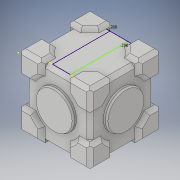
# Autodesk Inventor part: CapStone
Saved by Autodesk Inventor 2018 (Build 220112000, 112)
## iProperties
Created: 2020-01-09
Part Number: CapStone
Material: Generic
Document SubType Name: Modeling
Designer: AOFUser
Density: 1 g/cm^3
Appearance: Default
Author: AOFUser
Autodesk Inventor part; units mm, degrees
ref_plane "YZ Plane" through (0, 0, 0) normal (1, 0, 0) x (0, 1, 0)
ref_plane "XZ Plane" through (0, 0, 0) normal (0, 1, 0) x (-1, 0, 0)
ref_plane "XY Plane" through (0, 0, 0) normal (0, 0, 1) x (1, 0, 0)
sketch "Sketch1" plane through (0, 0, 0) normal (0, 1, 0) x (-1, 0, 0)
  line L0 (0, 0) -> (-101.6, 0)
  line L1 (-101.6, 0) -> (-101.6, -101.6)
  line L2 (-101.6, -101.6) -> (0, -101.6)
  line L3 (0, -101.6) -> (0, 0)
  dimension "d0" = 101.6
  dimension "d1" = 101.6
  constraints: 8 end point, 2 parallel, 1 horizontal, 1 perpendicular
  measures "d0" distance of L2.end L1.end
  measures "d1" distance of L1.end L0.end
extrude "Extrusion1" add sketch "Sketch1" along normal blind 101.6
sketch "Sketch2" plane through (101.6, 0, 0) normal (1, 0, 0) x (0, 0, -1)
  line L0 (0, 0) -> (33.02, 0)
  line L1 (0, 0) -> (101.6, 0) projected
  line L2 (0, 0) -> (0, 33.02)
  line L3 (0, 0) -> (0, 101.6) projected
  line L4 (0, 101.6) -> (0, 68.58)
  line L5 (0, 101.6) -> (33.02, 101.6)
  line L6 (0, 101.6) -> (101.6, 101.6) projected
  line L7 (101.6, 101.6) -> (68.58, 101.6)
  line L8 (101.6, 0) -> (101.6, 33.02)
  line L9 (101.6, 0) -> (101.6, 101.6) projected
  line L10 (101.6, 0) -> (68.58, 0)
  line L11 (33.02, 101.6) -> (68.58, 101.6)
  line L12 (68.58, 101.6) -> (68.58, 0)
  line L13 (68.58, 0) -> (33.02, 0)
  line L14 (33.02, 0) -> (33.02, 101.6)
  line L15 (0, 33.02) -> (101.6, 33.02)
  line L16 (101.6, 33.02) -> (101.6, 68.58)
  line L17 (101.6, 68.58) -> (0, 68.58)
  line L18 (0, 68.58) -> (0, 33.02)
  dimension "d4" = 33.02
  dimension "d5" = 33.02
  dimension "d6" = 33.02
  dimension "d7" = 33.02
  dimension "d8" = 33.02
  dimension "d9" = 33.02
  dimension "d10" = 33.02
  constraints: 30 end point, 8 point on line, 4 parallel, 2 horizontal, 2 perpendicular
  measures "d4" distance of L0.start L0.end
  measures "d5" distance of L0.start L2.end
  measures "d6" distance of L3.end L4.end
  measures "d7" distance of L3.end L5.end
  measures "d8" distance of L6.end L7.end
  measures "d9" distance of L1.end L8.end
  measures "d10" distance of L1.end L10.end
extrude "Extrusion2" cut sketch "Sketch2" against normal blind 5.08 contours L14 L15 L12 L1 | L3 L17 L14 L15 | L14 L17 L12 L15 | L12 L17 L9 L15 | L14 L6 L12 L17
sketch "Sketch3" plane through (101.6, 0, -101.6) normal (0, 0, -1) x (-1, 0, 0)
  line L0 (0, 0) -> (0, 33.02) projected
  line L1 (0, 0) -> (33.02, 0)
  line L2 (101.6, 0) -> (101.6, 101.6) projected
  line L3 (101.6, 0) -> (68.58, 0)
  line L4 (0, 0) -> (101.6, 0) projected
  line L5 (0, 101.6) -> (33.02, 101.6)
  line L6 (0, 101.6) -> (101.6, 101.6) projected
  line L7 (101.6, 101.6) -> (68.58, 101.6)
  line L8 (33.02, 0) -> (68.58, 0)
  line L9 (68.58, 0) -> (68.58, 101.6)
  line L10 (68.58, 101.6) -> (33.02, 101.6)
  line L11 (33.02, 101.6) -> (33.02, 0)
  line L12 (0, 68.58) -> (5.08, 68.58) projected
  line L13 (0, 68.58) -> (101.6, 68.58)
  line L14 (101.6, 68.58) -> (101.6, 33.02)
  line L15 (101.6, 33.02) -> (0, 33.02)
  line L16 (0, 33.02) -> (0, 68.58)
  dimension "d13" = 33.02
  dimension "d14" = 33.02
  dimension "d15" = 33.02
  dimension "d16" = 33.02
  constraints: 24 end point, 4 parallel, 4 point on line, 3 horizontal, 2 perpendicular
  measures "d13" distance of L0.start L1.end
  measures "d14" distance of L2.start L3.end
  measures "d15" distance of L5.start L5.end
  measures "d16" distance of L2.end L7.end
extrude "Extrusion3" cut sketch "Sketch3" against normal blind 5.08 contours L16 L12 L13 L11 L15 | L11 L15 L9 L4 | L11 L13 L9 L15 | L11 L6 L9 L13 | L9 L13 L2 L15
sketch "Sketch4" plane through (0, 0, -101.6) normal (-1, 0, 0) x (0, 0, 1)
  line L0 (33.02, 0) -> (0, 0) projected
  line L1 (0, 0) -> (33.02, 0)
  line L2 (33.02, 101.6) -> (0, 101.6) projected
  line L3 (-0.0001, 101.6) -> (33.02, 101.6)
  line L4 (101.6, 101.6) -> (68.58, 101.6) projected
  line L5 (101.6, 101.6) -> (68.58, 101.6)
  line L6 (101.6, 0) -> (101.6, 101.6) projected
  line L7 (101.6, 0) -> (68.58, 0)
  line L8 (0, 0) -> (101.6, 0) projected
  line L9 (68.58, 0) -> (68.58, 33.02) projected
  line L10 (33.02, 101.6) -> (68.58, 101.6)
  line L11 (68.58, 101.6) -> (68.58, 0)
  line L12 (68.58, 0) -> (33.02, 0)
  line L13 (33.02, 0) -> (33.02, 101.6)
  line L14 (33.02, 68.58) -> (0, 68.58) projected
  line L15 (101.6, 33.02) -> (101.6, 68.58) projected
  line L16 (0, 68.58) -> (101.6, 68.58)
  line L17 (101.6, 68.58) -> (101.6, 33.02)
  line L18 (101.6, 33.02) -> (0, 33.02)
  line L19 (0, 33.02) -> (0, 68.58)
  constraints: 24 end point, 4 parallel, 3 collinear, 2 horizontal, 2 perpendicular, 1 point on line
extrude "Extrusion4" cut sketch "Sketch4" against normal blind 5.08 contours L11 L16 L13 L10 | L6 L18 L11 L16 | L11 L18 L13 L16 | L13 L18 L19 L14 | L9 L8 L13 L18
sketch "Sketch5" plane through (0, 0, 0) normal (0, 0, 1) x (1, 0, 0)
  line L0 (0, 0) -> (0, 33.02) projected
  line L1 (33.02, 0) -> (0, 0) projected
  line L2 (0, 0) -> (33.02, 0)
  line L3 (0, 68.58) -> (0, 101.6) projected
  line L4 (33.02, 101.6) -> (33.02, 68.58) projected
  line L5 (0, 101.6) -> (33.02, 101.6)
  line L6 (68.58, 0) -> (68.58, 33.02) projected
  line L7 (33.02, 101.6) -> (68.58, 101.6)
  line L8 (68.58, 101.6) -> (68.58, 0)
  line L9 (68.58, 0) -> (33.02, 0)
  line L10 (33.02, 0) -> (33.02, 101.6)
  line L11 (101.6, 0) -> (101.6, 33.02) projected
  line L12 (0, 68.58) -> (101.6, 68.58)
  line L13 (101.6, 68.58) -> (101.6, 33.02)
  line L14 (101.6, 33.02) -> (0, 33.02)
  line L15 (0, 33.02) -> (0, 68.58)
  constraints: 20 end point, 5 equal length, 3 horizontal, 2 perpendicular
extrude "Extrusion5" cut sketch "Sketch5" against normal blind 5.08 contours L15 L12 L10 L14 | L10 L14 L6 L9 | L10 L12 L8 L14 | L4 L7 L8 L12 | L8 L12 L13 L14
sketch "Sketch6" plane through (0, 101.6, 0) normal (0, 1, 0) x (1, 0, 0)
  line L0 (68.58, 0) -> (101.6, 0) projected
  line L1 (68.58, 0) -> (33.02, 0)
  line L2 (33.02, 0) -> (33.02, 101.6)
  line L3 (33.02, 101.6) -> (68.58, 101.6)
  line L4 (68.58, 101.6) -> (68.58, 0)
  line L5 (101.6, 33.02) -> (101.6, 0) projected
  line L6 (0, 68.58) -> (5.08, 68.58) projected
  line L7 (101.6, 33.02) -> (0, 33.02)
  line L8 (0, 33.02) -> (0, 68.58)
  line L9 (0, 68.58) -> (101.6, 68.58)
  line L10 (101.6, 68.58) -> (101.6, 33.02)
  point P0 (0, 0)
  constraints: 16 end point, 4 parallel, 2 horizontal, 2 perpendicular
extrude "Extrusion6" cut sketch "Sketch6" against normal blind 5.08 contours L1 L2 L7 L4 | L7 L2 L9 L4 | L4 L9 L10 L7 | L7 L8 L6 L9 L2 | L9 L2 L3 L4
chamfer "Chamfer42" distance 5.08 distance2 5.08 1 edges at (5.08, 96.52, -50.8) measured on face at (5.08, 44.8733, -56.7267)
chamfer "Chamfer43" distance 5.08 distance2 5.08 1 edges at (50.8, 96.52, -96.52) measured on face at (44.8733, 44.8733, -96.52)
chamfer "Chamfer44" distance 5.08 distance2 5.08 1 edges at (96.52, 96.52, -50.8) measured on face at (96.52, 44.8733, -56.7267)
chamfer "Chamfer45" distance 5.08 distance2 5.08 1 edges at (50.8, 96.52, -5.08) measured on face at (56.7267, 44.8733, -5.08)
chamfer "Chamfer46" distance 5.08 distance2 5.08 1 edges at (5.08, 50.8, -96.52) measured on face at (44.8733, 44.8733, -96.52)
chamfer "Chamfer47" distance 5.08 distance2 5.08 1 edges at (5.08, 50.8, -5.08) measured on face at (5.08, 56.7267, -56.7267)
chamfer "Chamfer48" distance 5.08 distance2 5.08 1 edges at (5.08, 0, -50.8) measured on face at (56.7267, 0, -54.1867)
chamfer "Chamfer49" distance 5.08 distance2 5.08 1 edges at (50.8, 0, -96.52) measured on face at (38.9467, 0, -44.8733)
chamfer "Chamfer50" distance 5.08 distance2 5.08 1 edges at (50.8, 0, -5.08) measured on face at (58.42, 0, -52.4933)
chamfer "Chamfer51" distance 5.08 distance2 5.08 1 edges at (96.52, 0, -50.8) measured on face at (37.2533, 0, -56.7267)
chamfer "Chamfer52" distance 5.08 distance2 5.08 1 edges at (96.52, 50.8, -96.52) measured on face at (96.52, 44.8733, -56.7267)
chamfer "Chamfer53" distance 5.08 distance2 5.08 1 edges at (96.52, 50.8, -5.08) measured on face at (96.52, 44.8733, -44.8733)
chamfer "Chamfer54" distance 5.08 distance2 5.08 1 edges at (68.58, 101.6, -85.09) measured on face at (90.5933, 101.6, -79.5867)
chamfer "Chamfer55" distance 5.08 distance2 5.08 1 edges at (87.63, 101.6, -68.58) measured on face at (82.9733, 101.6, -90.5933)
chamfer "Chamfer56" distance 5.08 distance2 5.08 1 edges at (101.6, 101.6, -87.63) measured on face at (82.9733, 101.6, -92.2867)
chamfer "Chamfer57" distance 5.08 distance2 5.08 1 edges at (85.09, 101.6, -101.6) measured on face at (81.28, 101.6, -92.2867)
chamfer "Chamfer58" distance 5.08 distance2 5.08 1 edges at (68.58, 101.6, -16.51) measured on face at (90.5933, 101.6, -11.0067)
chamfer "Chamfer59" distance 5.08 distance2 5.08 1 edges at (87.63, 101.6, -33.02) measured on face at (92.2867, 101.6, -22.0133)
chamfer "Chamfer60" distance 5.08 distance2 5.08 1 edges at (87.63, 101.6, 0) measured on face at (82.9733, 101.6, -9.3133)
chamfer "Chamfer61" distance 5.08 distance2 5.08 1 edges at (101.6, 101.6, -16.51) measured on face at (92.2867, 101.6, -20.32)
chamfer "Chamfer62" distance 5.08 distance2 5.08 1 edges at (33.02, 101.6, -16.51) measured on face at (22.0133, 101.6, -22.0133)
chamfer "Chamfer63" distance 5.08 distance2 5.08 1 edges at (0, 101.6, -16.51) measured on face at (18.6267, 101.6, -22.0133)
chamfer "Chamfer64" distance 5.08 distance2 5.08 1 edges at (16.51, 101.6, 0) measured on face at (20.32, 101.6, -22.0133)
chamfer "Chamfer65" distance 5.08 distance2 5.08 1 edges at (16.51, 101.6, -33.02) measured on face at (20.32, 101.6, -23.7067)
chamfer "Chamfer66" distance 5.08 distance2 5.08 1 edges at (33.02, 101.6, -85.09) measured on face at (11.0067, 101.6, -90.5933)
chamfer "Chamfer67" distance 5.08 distance2 5.08 1 edges at (13.97, 101.6, -68.58) measured on face at (9.3133, 101.6, -90.5933)
chamfer "Chamfer68" distance 5.08 distance2 5.08 1 edges at (13.97, 101.6, -101.6) measured on face at (9.3133, 101.6, -82.9733)
chamfer "Chamfer69" distance 5.08 distance2 5.08 1 edges at (0, 101.6, -85.09) measured on face at (9.3133, 101.6, -88.9)
chamfer "Chamfer70" distance 5.08 distance2 5.08 1 edges at (101.6, 16.51, 0) measured on face at (79.5867, 11.0067, 0)
chamfer "Chamfer71" distance 5.08 distance2 5.08 1 edges at (101.6, 16.51, -33.02) measured on face at (101.6, 22.0133, -23.7067)
chamfer "Chamfer72" distance 5.08 distance2 5.08 1 edges at (101.6, 68.58, -16.51) measured on face at (101.6, 77.8933, -11.0067)
chamfer "Chamfer73" distance 5.08 distance2 5.08 1 edges at (101.6, 85.09, -33.02) measured on face at (101.6, 81.28, -11.0067)
chamfer "Chamfer74" distance 5.08 distance2 5.08 1 edges at (101.6, 85.09, 0) measured on face at (77.8933, 77.8933, 0)
chamfer "Chamfer75" distance 5.08 distance2 5.08 1 edges at (101.6, 82.55, -68.58) measured on face at (101.6, 77.8933, -79.5867)
chamfer "Chamfer76" distance 5.08 distance2 5.08 1 edges at (101.6, 82.55, -101.6) measured on face at (101.6, 87.2067, -92.2867)
chamfer "Chamfer77" distance 5.08 distance2 5.08 1 edges at (101.6, 68.58, -85.09) measured on face at (101.6, 87.2067, -88.9)
chamfer "Chamfer78" distance 5.08 distance2 5.08 1 edges at (101.6, 16.51, -68.58) measured on face at (101.6, 11.0067, -79.5867)
chamfer "Chamfer79" distance 5.08 distance2 5.08 1 edges at (101.6, 16.51, -101.6) measured on face at (101.6, 11.0067, -82.9733)
chamfer "Chamfer80" distance 5.08 distance2 5.08 1 edges at (101.6, 33.02, -85.09) measured on face at (101.6, 22.0133, -81.28)
chamfer "Chamfer81" distance 5.08 distance2 5.08 1 edges at (101.6, 33.02, -16.51) measured on face at (101.6, 22.0133, -20.32)
chamfer "Chamfer82" distance 5.08 distance2 5.08 1 edges at (101.6, 0, -16.51) measured on face at (101.6, 9.3133, -12.7)
chamfer "Chamfer83" distance 5.08 distance2 5.08 1 edges at (82.55, 0, 0) measured on face at (87.2067, 22.0133, 0)
chamfer "Chamfer84" distance 5.08 distance2 5.08 1 edges at (16.51, 0, 0) measured on face at (22.0133, 22.0133, 0)
chamfer "Chamfer85" distance 5.08 distance2 5.08 1 edges at (0, 0, -19.05) measured on face at (0, 23.7067, -11.0067)
chamfer "Chamfer86" distance 5.08 distance2 5.08 1 edges at (0, 0, -85.09) measured on face at (0, 22.0133, -90.5933)
chamfer "Chamfer87" distance 5.08 distance2 5.08 1 edges at (19.05, 0, -101.6) measured on face at (11.0067, 23.7067, -101.6)
chamfer "Chamfer88" distance 5.08 distance2 5.08 1 edges at (82.55, 0, -101.6) measured on face at (77.8933, 22.0133, -101.6)
chamfer "Chamfer89" distance 5.08 distance2 5.08 1 edges at (101.6, 0, -85.09) measured on face at (101.6, 9.3133, -81.28)
chamfer "Chamfer90" distance 5.08 distance2 5.08 1 edges at (0, 82.55, 0) measured on face at (0, 77.8933, -22.0133)
chamfer "Chamfer91" distance 5.08 distance2 5.08 1 edges at (0, 82.55, -33.02) measured on face at (0, 77.8933, -23.7067)
chamfer "Chamfer92" distance 5.08 distance2 5.08 1 edges at (0, 82.55, -68.58) measured on face at (0, 87.2067, -90.5933)
chamfer "Chamfer93" distance 5.08 distance2 5.08 1 edges at (0, 82.55, -101.6) measured on face at (22.0133, 77.8933, -101.6)
chamfer "Chamfer94" distance 5.08 distance2 5.08 1 edges at (0, 68.58, -85.09) measured on face at (0, 87.2067, -81.28)
chamfer "Chamfer95" distance 5.08 distance2 5.08 1 edges at (0, 68.58, -16.51) measured on face at (0, 87.2067, -12.7)
chamfer "Chamfer96" distance 5.08 distance2 5.08 1 edges at (0, 33.02, -16.51) measured on face at (0, 14.3933, -22.0133)
chamfer "Chamfer97" distance 5.08 distance2 5.08 1 edges at (0, 16.51, -33.02) measured on face at (0, 12.7, -22.0133)
chamfer "Chamfer98" distance 5.08 distance2 5.08 1 edges at (0, 16.51, 0) measured on face at (0, 20.32, -9.3133)
chamfer "Chamfer99" distance 5.08 distance2 5.08 1 edges at (0, 19.05, -68.58) measured on face at (0, 14.3933, -90.5933)
chamfer "Chamfer100" distance 5.08 distance2 5.08 1 edges at (0, 19.05, -101.6) measured on face at (22.0133, 14.3933, -101.6)
chamfer "Chamfer101" distance 5.08 distance2 5.08 1 edges at (0, 33.02, -85.09) measured on face at (0, 23.7067, -88.9)
chamfer "Chamfer102" distance 5.08 distance2 5.08 1 edges at (33.02, 82.55, 0) measured on face at (14.3933, 77.8933, 0)
chamfer "Chamfer103" distance 5.08 distance2 5.08 1 edges at (16.51, 68.58, 0) measured on face at (12.7, 77.8933, 0)
chamfer "Chamfer104" distance 5.08 distance2 5.08 1 edges at (82.55, 68.58, 0) measured on face at (77.8933, 87.2067, 0)
chamfer "Chamfer105" distance 5.08 distance2 5.08 1 edges at (68.58, 85.09, 0) measured on face at (77.8933, 81.28, 0)
chamfer "Chamfer106" distance 5.08 distance2 5.08 1 edges at (19.05, 33.02, 0) measured on face at (23.7067, 23.7067, 0)
chamfer "Chamfer107" distance 5.08 distance2 5.08 1 edges at (33.02, 16.51, 0) measured on face at (23.7067, 12.7, 0)
chamfer "Chamfer108" distance 5.08 distance2 5.08 1 edges at (68.58, 19.05, 0) measured on face at (77.8933, 23.7067, 0)
chamfer "Chamfer109" distance 5.08 distance2 5.08 1 edges at (85.09, 33.02, 0) measured on face at (81.28, 23.7067, 0)
chamfer "Chamfer110" distance 5.08 distance2 5.08 1 edges at (68.58, 82.55, -101.6) measured on face at (87.2067, 87.2067, -101.6)
chamfer "Chamfer111" distance 5.08 distance2 5.08 1 edges at (33.02, 82.55, -101.6) measured on face at (23.7067, 87.2067, -101.6)
chamfer "Chamfer112" distance 5.08 distance2 5.08 1 edges at (85.09, 68.58, -101.6) measured on face at (88.9, 87.2067, -101.6)
chamfer "Chamfer113" distance 5.08 distance2 5.08 1 edges at (16.51, 68.58, -101.6) measured on face at (12.7, 87.2067, -101.6)
chamfer "Chamfer114" distance 5.08 distance2 5.08 1 edges at (82.55, 33.02, -101.6) measured on face at (77.8933, 23.7067, -101.6)
chamfer "Chamfer115" distance 5.08 distance2 5.08 1 edges at (68.58, 16.51, -101.6) measured on face at (77.8933, 20.32, -101.6)
chamfer "Chamfer116" distance 5.08 distance2 5.08 1 edges at (19.05, 33.02, -101.6) measured on face at (23.7067, 14.3933, -101.6)
chamfer "Chamfer117" distance 5.08 distance2 5.08 1 edges at (33.02, 16.51, -101.6) measured on face at (23.7067, 12.7, -101.6)
sketch "Sketch9" plane through (101.6, 0, -96.52) normal (0, 0, -1) x (-1, 0, 0)
  line L0 (68.58, 96.52) -> (33.02, 96.52) projected
  line L1 (50.8, 96.52) -> (50.8, 0)
  line L2 (33.02, 0) -> (68.58, 0) projected
  line L3 (5.08, 33.02) -> (5.08, 68.58) projected
  line L4 (5.08, 50.8) -> (96.52, 50.8)
  line L5 (96.52, 68.58) -> (96.52, 33.02) projected
  circle A0 centre (50.8, 50.8) radius 35.56
  point P0 (101.6, 0)
  dimension "d376" = 71.12
  constraints: 5 midpoint, 4 end point, 1 centre point
  measures "d376" diameter of A0
extrude "Extrusion7" cut sketch "Sketch9" along normal blind 5.08
sketch "Sketch11" plane through (5.08, 0, -101.6) normal (-1, 0, 0) x (0, 0, 1)
  line L0 (33.02, 96.52) -> (68.58, 96.52) projected
  line L1 (50.8, 96.52) -> (50.8, 0)
  line L2 (33.02, 0) -> (68.58, 0) projected
  line L3 (5.08, 68.58) -> (5.08, 33.02) projected
  line L4 (5.08, 50.8) -> (96.52, 50.8)
  line L5 (96.52, 68.58) -> (96.52, 33.02) projected
  circle A0 centre (50.8, 50.8) radius 35.56
  point P0 (101.6, 0)
  dimension "d379" = 71.12
  constraints: 5 midpoint, 4 end point, 1 centre point
  measures "d379" diameter of A0
extrude "Extrusion8" cut sketch "Sketch11" along normal blind 5.08
sketch "Sketch12" plane through (0, 0, -5.08) normal (0, 0, 1) x (1, 0, 0)
  line L0 (68.58, 96.52) -> (33.02, 96.52) projected
  line L1 (50.8, 96.52) -> (50.8, 0)
  line L2 (5.08, 68.58) -> (5.08, 33.02) projected
  line L3 (5.08, 50.8) -> (96.3319, 50.8)
  circle A0 centre (50.7059, 50.8) radius 35.56
  point P0 (0, 0)
  dimension "d382" = 71.12
  constraints: 4 end point, 3 midpoint, 1 centre point, 1 horizontal, 1 vertical
  measures "d382" diameter of A0
extrude "Extrusion9" cut sketch "Sketch12" along normal blind 5.08
sketch "Sketch13" plane through (96.52, 0, 0) normal (1, 0, 0) x (0, 0, -1)
  line L0 (33.02, 96.52) -> (68.58, 96.52) projected
  line L1 (50.8, 96.52) -> (50.8, 0)
  line L2 (68.58, 0) -> (33.02, 0) projected
  line L3 (5.08, 33.02) -> (5.08, 68.58) projected
  line L4 (5.08, 50.8) -> (96.52, 50.8)
  line L5 (96.52, 68.58) -> (96.52, 33.02) projected
  circle A0 centre (50.8, 50.8) radius 35.56
  point P0 (0, 0)
  dimension "d385" = 71.12
  constraints: 5 midpoint, 4 end point, 1 centre point
  measures "d385" diameter of A0
extrude "Extrusion10" cut sketch "Sketch13" along normal blind 5.08
chamfer "Chamfer118" distance 5.08 distance2 5.08 1 edges at (101.6, 75.9447, -25.6553) measured on face at (101.6, 89.9016, -19.8055)
chamfer "Chamfer119" distance 5.08 distance2 5.08 1 edges at (101.6, 75.9447, -75.9447) measured on face at (101.6, 81.7945, -89.9016)
chamfer "Chamfer120" distance 5.08 distance2 5.08 1 edges at (101.6, 25.6553, -75.9447) measured on face at (101.6, 19.8055, -89.9016)
chamfer "Chamfer121" distance 5.08 distance2 5.08 1 edges at (101.6, 25.6553, -25.6553) measured on face at (101.6, 11.6984, -19.8055)
chamfer "Chamfer122" distance 5.08 distance2 5.08 1 edges at (75.9447, 75.9447, -101.6) measured on face at (81.7945, 89.9016, -101.6)
chamfer "Chamfer123" distance 5.08 distance2 5.08 1 edges at (25.6553, 75.9447, -101.6) measured on face at (11.6984, 81.7945, -101.6)
chamfer "Chamfer124" distance 5.08 distance2 5.08 1 edges at (25.6553, 25.6553, -101.6) measured on face at (11.6984, 19.8055, -101.6)
chamfer "Chamfer125" distance 5.08 distance2 5.08 1 edges at (75.9447, 25.6553, -101.6) measured on face at (81.7945, 11.6984, -101.6)
chamfer "Chamfer126" distance 5.08 distance2 5.08 1 edges at (0, 75.9447, -75.9447) measured on face at (0, 89.9016, -81.7945)
chamfer "Chamfer127" distance 5.08 distance2 5.08 1 edges at (0, 75.9447, -25.6553) measured on face at (0, 81.7945, -11.6984)
chamfer "Chamfer128" distance 5.08 distance2 5.08 1 edges at (0, 25.6553, -75.9447) measured on face at (0, 11.6984, -81.7945)
chamfer "Chamfer129" distance 5.08 distance2 5.08 1 edges at (0, 25.6553, -25.6553) measured on face at (0, 19.8055, -11.6984)
chamfer "Chamfer130" distance 5.08 distance2 5.08 1 edges at (25.6046, 75.988, 0) measured on face at (19.794, 89.9202, 0)
chamfer "Chamfer131" distance 5.08 distance2 5.08 1 edges at (75.8941, 75.9012, 0) measured on face at (89.8796, 81.7846, 0)
chamfer "Chamfer132" distance 5.08 distance2 5.08 1 edges at (75.8941, 25.6988, 0) measured on face at (89.8796, 19.8154, 0)
chamfer "Chamfer133" distance 5.08 distance2 5.08 1 edges at (25.6046, 25.612, 0) measured on face at (19.794, 11.6798, 0)
sketch "Sketch14" plane through (0, 96.52, 0) normal (0, 1, 0) x (1, 0, 0)
  line L0 (33.02, 5.08) -> (68.58, 5.08) projected
  line L1 (50.8, 5.08) -> (50.8, 96.52)
  line L2 (68.58, 96.52) -> (33.02, 96.52) projected
  line L3 (96.52, 33.02) -> (96.52, 68.58) projected
  line L4 (96.52, 50.8) -> (5.08, 50.8)
  line L5 (5.08, 68.58) -> (5.08, 33.02) projected
  circle A0 centre (50.8, 50.8) radius 35.56
  point P0 (0, 0)
  dimension "d436" = 71.12
  constraints: 5 midpoint, 4 end point, 1 centre point
  measures "d436" diameter of A0
extrude "Extrusion11" cut sketch "Sketch14" along normal blind 5.08
chamfer "Chamfer134" distance 5.08 distance2 5.08 1 edges at (75.9447, 101.6, -25.6553) measured on face at (89.9016, 101.6, -19.8055)
chamfer "Chamfer135" distance 5.08 distance2 5.08 1 edges at (25.6553, 101.6, -25.6553) measured on face at (19.8055, 101.6, -11.6984)
chamfer "Chamfer136" distance 5.08 distance2 5.08 1 edges at (75.9447, 101.6, -75.9447) measured on face at (89.9016, 101.6, -81.7945)
chamfer "Chamfer137" distance 5.08 distance2 5.08 1 edges at (25.6553, 101.6, -75.9447) measured on face at (19.8055, 101.6, -89.9016)
sketch "Sketch15" plane through (96.52, 0, 0) normal (1, 0, 0) x (0, 0, -1)
  line L0 (5.08, 68.58) -> (5.08, 33.02) projected
  line L1 (5.08, 50.8) -> (96.52, 50.8)
  line L2 (96.52, 68.58) -> (96.52, 33.02) projected
  line L3 (33.02, 96.52) -> (68.58, 96.52) projected
  line L4 (50.8, 96.52) -> (50.8, 0)
  circle A0 centre (50.8, 50.8) radius 26.67
  point P0 (0, 0)
  dimension "d451" = 53.34
  constraints: 4 end point, 4 midpoint, 1 centre point, 1 point on line, 1 vertical
  measures "d451" diameter of A0
extrude "Extrusion12" add sketch "Sketch15" along normal blind 5.08
sketch "Sketch16" plane through (101.6, 0, -96.52) normal (0, 0, -1) x (-1, 0, 0)
  line L0 (68.58, 96.52) -> (33.02, 96.52) projected
  line L1 (50.8, 96.52) -> (50.8, 0)
  line L2 (5.08, 33.02) -> (5.08, 68.58) projected
  line L3 (5.08, 50.8) -> (96.52, 50.8)
  line L4 (96.52, 68.58) -> (96.52, 33.02) projected
  circle A0 centre (50.8, 50.8) radius 26.67
  point P0 (101.6, 0)
  dimension "d454" = 53.34
  constraints: 4 end point, 4 midpoint, 1 centre point, 1 vertical
  measures "d454" diameter of A0
sketch "Sketch17" plane through (5.08, 0, -101.6) normal (-1, 0, 0) x (0, 0, 1)
  circle A0 centre (50.8, 50.8) radius 26.67 projected
  circle A1 centre (50.8, 50.8) radius 26.67
  point P0 (101.6, 0)
  dimension "d455" = 53.34
  constraints: 1 centre point, 1 coincident
  measures "d455" diameter of A1
sketch "Sketch18" plane through (0, 0, -5.08) normal (0, 0, 1) x (1, 0, 0)
  line L0 (33.02, 96.52) -> (68.58, 96.52) projected
  line L1 (50.8, 96.52) -> (50.8, 0)
  line L2 (5.08, 68.58) -> (5.08, 33.02) projected
  line L3 (5.08, 50.8) -> (101.4002, 50.8)
  circle A0 centre (50.8, 50.8) radius 26.67
  point P0 (0, 0)
  dimension "d456" = 53.34
  constraints: 4 end point, 2 midpoint, 2 point on line, 1 centre point, 1 horizontal, 1 vertical
  measures "d456" diameter of A0
extrude "Extrusion13" add sketch "Sketch18" along normal blind 5.08
extrude "Extrusion14" add sketch "Sketch17" along normal blind 5.08
extrude "Extrusion15" add sketch "Sketch16" along normal blind 5.08
chamfer "Chamfer138" distance 1.27 distance2 2.54 1 edges at (24.13, 50.8, 0) measured on face at (47.893, 58.1163, 0)
chamfer "Chamfer139" distance 1.27 distance2 2.54 1 edges at (0, 50.8, -77.47) measured on face at (0, 58.1163, -53.707)
chamfer "Chamfer140" distance 1.27 distance2 2.54 1 edges at (77.47, 50.8, -101.6) measured on face at (53.707, 58.1163, -101.6)
chamfer "Chamfer141" distance 1.27 distance2 2.54 1 edges at (101.6, 50.8, -24.13) measured on face at (101.6, 58.1163, -47.893)
sketch "Sketch19" plane through (0, 96.52, 0) normal (0, 1, 0) x (1, 0, 0)
  line L0 (33.02, 91.44) -> (33.02, 96.52) projected
  line L1 (33.02, 91.44) -> (38.1, 91.44)
  line L2 (68.58, 91.44) -> (33.02, 91.44) projected
  line L3 (68.58, 91.44) -> (63.5, 91.44)
  line L4 (68.58, 10.16) -> (33.02, 10.16) projected
  line L5 (38.1, 91.44) -> (63.5, 91.44)
  line L6 (63.5, 91.44) -> (63.5, 10.16)
  line L7 (63.5, 10.16) -> (38.1, 10.16)
  line L8 (38.1, 10.16) -> (38.1, 91.44)
  point P0 (0, 0)
  dimension "d475" = 5.08
  dimension "d476" = 5.08
  constraints: 12 end point, 3 point on line, 2 parallel, 1 horizontal, 1 perpendicular
  measures "d475" distance of L0.start L1.end
  measures "d476" distance of L2.start L3.end
body "Solid1"
